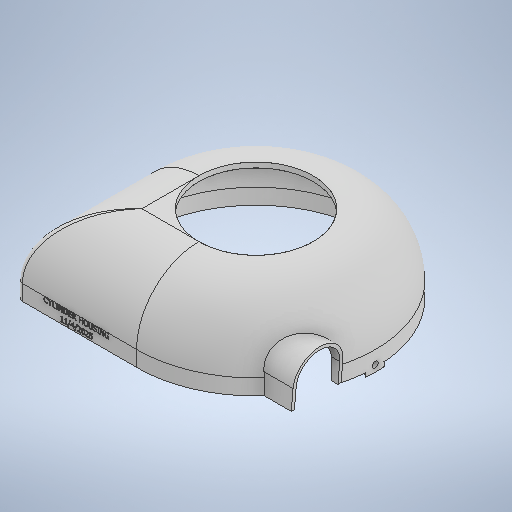
# Autodesk Inventor part: Cylinder Housing_cap_3
Saved by Autodesk Inventor 2025 (Build 290162000, 162)
## iProperties
Created: 2025-10-06
Part Number: Cylinder Housing_cap_3
Material: Generic
Document SubType Name: Modeling
Designer: mumin
Density: 1 g/cm^3
Appearance: Default
Author: mumin
Autodesk Inventor part; units mm, degrees
ref_plane "XZ Plane" through (0, 0, 0) normal (0, 1, 0) x (-1, 0, 0)
ref_plane "XY Plane" through (0, 0, 0) normal (0, 0, 1) x (1, 0, 0)
sketch "Sketch1" plane through (0, 0, 0) normal (0, 1, 0) x (-1, 0, 0)
  arc A0 (0, 115) -> (115, 0) centre (0, 0) ccw
  line L0 (115, 0) -> (115, 110)
  line L1 (110, 115) -> (0, 115)
  arc A1 (115, 110) -> (110, 115) centre (110, 110) ccw
  dimension "d0" = 230
  dimension "d1" = 5
  constraints: 4 end point, 4 point on circle, 2 centre point, 2 tangent, 1 coincident
  measures "d0" diameter of A0
  measures "d1" radius of A1
extrude "Base Shape & Wall" add sketch "Sketch1" along normal blind 75
fillet "Curved Edge" radius 60 4 edges at (81.3173, 75, -81.3173) (-115, 75, 55) (-113.5355, 75, 113.5355) (-55, 75, 115)
shell "Shell" thickness 4.9 removed faces 1 at (-52.6749, 0, -2.0856)
sketch "Sketch2" plane through (0, 75, 0) normal (0, 1, 0) x (1, 0, 0)
  point P0 (0, 0)
  point P1 (0, 0)
  constraints: 1 coincident
hole "Cylinder Hole" at (0, 75, 0) direction (0, -1, 0) diameter 109.9 end through all
sketch "Sketch3" plane through (0, 0, 0) normal (0, -1, 0) x (1, 0, 0)
  arc A0 (-115, 0) -> (0, 115) centre (0, 0) ccw projected
  line L0 (0, 55) -> (0, 110.1) projected
  line L1 (-110.1, 0) -> (-55, 0) projected
  arc A1 (-110.1, 0) -> (0, 110.1) centre (0, 0) ccw projected
  line L2 (114.6551, 8.9) -> (109.9418, 5.9)
  line L3 (109.9418, -5.9) -> (114.6551, -8.9)
  line L4 (-199.1076, 0) -> (222.9249, 0) projected
  arc A2 (-55, 0) -> (0, 55) centre (0, 0) ccw projected
  dimension "d13" = 5.9
  dimension "d14" = 8.9
  constraints: 4 end point, 4 point on circle, 2 symmetric about line
  measures "d13" distance from line of L4 L2.end
  measures "d14" distance from line of L4 L2.start
extrude "Front Tab" add sketch "Sketch3" along normal blind 4 contours L3 A1 L4 A0 | L4 A1 L2 A0 picked at (113.1479, -6.9122)
sketch "Sketch4" plane through (0, 0, 0) normal (1, 0, 0) x (0, 1, 0)
  line L0 (0, 0) -> (15, 0) projected
  circle A0 centre (2.5, 0) radius 2.75
  line L1 (-4, 8.9) -> (-4, -8.9) projected
  dimension "d17" = 5.5
  dimension "d18" = 6.5
  constraints: 1 centre point, 1 point on line
  measures "d17" diameter of A0
  measures "d18" distance from line of L1 A0.centre
extrude "Bolt Hole" cut sketch "Sketch4" along normal through all
sketch "Sketch5" plane through (0, 0, 0) normal (0, 0, 1) x (1, 0, 0)
  line L0 (-110.1, 0) -> (-108.0437, 0)
  line L1 (-110.1, 0) -> (-110.1, 15) projected
  line L2 (-110.1, 0) -> (-110.1, 10.1)
  line L3 (-110.1, 10.1) -> (-113.1, 10.1)
  line L4 (-113.1, 10.1) -> (-110.1, 0)
  line L5 (-109.0719, 10.1) -> (-109.0719, 0)
  line L6 (-110.1, 10.1) -> (-109.0719, 10.1)
  point P0 (0, 0)
  point P1 (0, 15)
  dimension "d43" = 10.1
  dimension "d44" = 3
  constraints: 12 end point, 2 horizontal, 1 midpoint, 1 perpendicular, 1 point on line
  measures "d43" distance of L0.start L2.end
  measures "d44" distance of L2.end L3.end
extrude "Hinge Tab Recess" cut sketch "Sketch5" along normal mid plane 15
sketch "Sketch6" plane through (0, 0, 0) normal (1, 0, 0) x (0, 1, 0)
  arc A0 (20, 32.226) -> (20, 74.226) centre (20, 53.226) ccw
  line L0 (0, 8.9) -> (0, 115) projected
  line L1 (20, 74.226) -> (0, 74.226)
  line L2 (0, 74.226) -> (0, 32.226)
  line L3 (0, 32.226) -> (20, 32.226)
  point P0 (0, 0)
  dimension "d25" = 42
  dimension "d26" = 53.226
  dimension "d27" = 20
  constraints: 6 end point, 2 point on circle, 1 centre point, 1 horizontal, 1 parallel, 1 perpendicular, 1 point on line
  measures "d25" diameter of A0
  measures "d26" vertical distance of point (0, 0) A0.centre
  measures "d27" distance from line of L0 A0.centre
extrude "LV Hole" cut sketch "Sketch6" along normal through all
ref_plane "Work Plane1" through (115, 0, 0) normal (1, 0, 0) x (0, 1, 0)
sketch "Sketch8" plane through (115, 0, 0) normal (1, 0, 0) x (0, 1, 0)
  spline S0 degree 5 poles (20, 74.226) (21.7452, 74.226) (23.5079, 74.045) (25.2552, 73.6747) (26.9529, 73.1202) (29.9438, 71.784) (31.2609, 71.0468) (32.4954, 70.2012) (33.6326, 69.2644) (35.8574, 67.094) (36.9093, 65.8358) (37.811, 64.5157) (38.5629, 63.1597) (39.9244, 60.1101) (40.4634, 58.4091) (40.8112, 56.7153) (40.9848, 55.0472) (41.0281, 50.1315) (40.4151, 46.9848) (39.2704, 44.0382) (37.5933, 41.2886) (34.2813, 37.7546) (33.1162, 36.7127) (31.8193, 35.7519) (30.3873, 34.8935) (28.01, 33.793) (27.1625, 33.4531) (26.2801, 33.1539) (25.3653, 32.9001) (23.9884, 32.6034) (23.5482, 32.5207) (23.1027, 32.4491) (22.6524, 32.3892) (21.7638, 32.2956) (21.3262, 32.261) (20.8833, 32.2376) (20.4431, 32.226) (20, 32.226) knots 0 0 0 0 0 0 0.115277 0.115277 0.115277 0.115277 0.213785 0.213785 0.213785 0.213785 0.327655 0.327655 0.327655 0.327655 0.466839 0.466839 0.466839 0.466839 0.745876 0.745876 0.745876 0.745876 0.873844 0.873844 0.873844 0.873844 0.940211 0.940211 0.940211 0.940211 0.970786 0.970786 0.970786 0.970786 1 1 1 1 1 1 projected
  line L0 (15, 74.226) -> (20, 74.226) projected
  line L1 (0, 74.226) -> (15, 74.226) projected
  line L2 (20, 32.226) -> (15, 32.226) projected
  line L3 (15, 32.226) -> (0, 32.226) projected
  line L4 (0, 29.226) -> (15, 29.226)
  line L5 (15, 29.226) -> (20, 29.226)
  line L6 (20, 77.226) -> (15, 77.226)
  line L7 (15, 77.226) -> (0, 77.226)
  line L8 (0, 77.226) -> (0, 74.226)
  line L9 (0, 0) -> (0, 110) projected
  line L10 (0, 32.226) -> (0, 29.226)
  spline S1 degree 5 poles (20, 29.226) (24.9777, 29.2263) (29.9563, 30.5154) (34.4863, 33.1008) (41.4168, 40.0057) (44.3283, 49.2848) (44.6352, 53.9403) (42.8551, 64.1602) (36.1874, 72.3028) (31.2207, 75.5896) (25.6093, 77.2254) (20, 77.226) knots 0 0 0 0 0 0 0.330105 0.330105 0.330105 0.628 0.628 0.628 1 1 1 1 1 1
  dimension "d38" = 3
  constraints: 12 end point, 2 collinear, 2 parallel, 2 vertical alignment, 4 other
extrude "LV Hood" add sketch "Sketch8" against normal up to surface contours L0 L1 L8 L7 L6 S1 L5 L4 L9 L3 L2 S0
sketch "Sketch9" plane through (115, 0, 77.226) normal (0, 0, 1) x (1, 0, 0)
  line L0 (-3.7757, 15) -> (-3.7757, 0) projected
  line L1 (0, 20) -> (-3.9915, 20) projected
  line L2 (0, 0) -> (0, 20) projected
  line L3 (0, 0) -> (-3.7757, 0) projected
  line L4 (0, 20) -> (0, 44) projected
  line L5 (-3.7757, 0) -> (0, 44)
  line L6 (0, 44) -> (0, 0)
  point P0 (-115, 0)
  constraints: 4 end point, 1 collinear, 1 other
extrude "Hood Slant Cut" cut sketch "Sketch9" against normal up to surface (48 mm away)
fillet "Fillet2" radius 0.2 1 edges at (-113.1, 10.1, 0)
sketch "Sketch10" plane through (-110, 0, 115) normal (0, 0, 1) x (1, 0, 0)
  line L0 (20.3517, 14.9708) -> (83.5486, 14.9708) construction
  line L1 (83.5486, 14.9708) -> (83.5486, 0.5472) construction
  line L2 (83.5486, 0.5472) -> (20.3517, 0.5472) construction
  line L3 (20.3517, 0.5472) -> (20.3517, 14.9708) construction
  spline S0 degree 2 poles (22.8112, 9.7763) (22.325, 9.7763) (21.5024, 10.1045) (21.2026, 10.4327) knots 0 0 0 1 2 2 2
  spline S1 degree 2 poles (21.2026, 10.4327) (20.9028, 10.7569) (20.5746, 11.7293) (20.5746, 12.3614) knots 0 0 0 1 2 2 2
  spline S2 degree 2 poles (20.5746, 12.3614) (20.5746, 12.9895) (20.8947, 13.9214) (21.1985, 14.2658) knots 0 0 0 1 2 2 2
  spline S3 degree 2 poles (21.1985, 14.2658) (21.4984, 14.6021) (22.3169, 14.9546) (22.8233, 14.9546) knots 0 0 0 1 2 2 2
  spline S4 degree 2 poles (22.8233, 14.9546) (23.0746, 14.9546) (23.5162, 14.8817) (23.7026, 14.825) knots 0 0 0 1 2 2 2
  spline S5 degree 2 poles (23.7026, 14.825) (23.8647, 14.7723) (24.201, 14.6224) (24.3671, 14.5332) knots 0 0 0 1 2 2 2
  line L4 (24.3671, 14.5332) -> (24.3671, 13.7309)
  line L5 (24.3671, 13.7309) -> (24.3144, 13.7309)
  spline S6 degree 2 poles (24.3144, 13.7309) (24.2253, 13.812) (23.9498, 14.0389) (23.7512, 14.1483) knots 0 0 0 1 2 2 2
  spline S7 degree 2 poles (23.7512, 14.1483) (23.5608, 14.2536) (23.111, 14.3873) (22.8193, 14.3873) knots 0 0 0 1 2 2 2
  spline S8 degree 2 poles (22.8193, 14.3873) (22.4992, 14.3873) (21.9279, 14.124) (21.7131, 13.8728) knots 0 0 0 1 2 2 2
  spline S9 degree 2 poles (21.7131, 13.8728) (21.5024, 13.6175) (21.2674, 12.8436) (21.2674, 12.3614) knots 0 0 0 1 2 2 2
  spline S10 degree 2 poles (21.2674, 12.3614) (21.2674, 11.8468) (21.5146, 11.1053) (21.7293, 10.8501) knots 0 0 0 1 2 2 2
  spline S11 degree 2 poles (21.7293, 10.8501) (21.94, 10.6029) (22.5032, 10.3517) (22.8193, 10.3517) knots 0 0 0 1 2 2 2
  spline S12 degree 2 poles (22.8193, 10.3517) (23.107, 10.3517) (23.5972, 10.4935) (23.7877, 10.5989) knots 0 0 0 1 2 2 2
  spline S13 degree 2 poles (23.7877, 10.5989) (23.97, 10.7042) (24.2415, 10.923) (24.3185, 11) knots 0 0 0 1 2 2 2
  line L6 (24.3185, 11) -> (24.3671, 11)
  line L7 (24.3671, 11) -> (24.3671, 10.2058)
  spline S14 degree 2 poles (24.3671, 10.2058) (24.201, 10.1288) (23.9092, 9.987) (23.7026, 9.9222) knots 0 0 0 1 2 2 2
  spline S15 degree 2 poles (23.7026, 9.9222) (23.4838, 9.8493) (23.111, 9.7763) (22.8112, 9.7763) knots 0 0 0 1 2 2 2
  line L8 (28.4878, 14.8655) -> (26.7982, 12.0778)
  line L9 (26.7982, 12.0778) -> (26.7982, 9.8655)
  line L10 (26.7982, 9.8655) -> (26.1337, 9.8655)
  line L11 (26.1337, 9.8655) -> (26.1337, 12.0089)
  line L12 (26.1337, 12.0089) -> (24.4441, 14.8655)
  line L13 (24.4441, 14.8655) -> (25.1815, 14.8655)
  line L14 (25.1815, 14.8655) -> (26.4741, 12.6653)
  line L15 (26.4741, 12.6653) -> (27.7828, 14.8655)
  line L16 (27.7828, 14.8655) -> (28.4878, 14.8655)
  line L17 (31.8468, 9.8655) -> (28.9498, 9.8655)
  line L18 (28.9498, 9.8655) -> (28.9498, 14.8655)
  line L19 (28.9498, 14.8655) -> (29.6143, 14.8655)
  line L20 (29.6143, 14.8655) -> (29.6143, 10.457)
  line L21 (29.6143, 10.457) -> (31.8468, 10.457)
  line L22 (31.8468, 10.457) -> (31.8468, 9.8655)
  line L23 (34.1118, 9.8655) -> (32.175, 9.8655)
  line L24 (32.175, 9.8655) -> (32.175, 10.376)
  line L25 (32.175, 10.376) -> (32.8112, 10.376)
  line L26 (32.8112, 10.376) -> (32.8112, 14.3549)
  line L27 (32.8112, 14.3549) -> (32.175, 14.3549)
  line L28 (32.175, 14.3549) -> (32.175, 14.8655)
  line L29 (32.175, 14.8655) -> (34.1118, 14.8655)
  line L30 (34.1118, 14.8655) -> (34.1118, 14.3549)
  line L31 (34.1118, 14.3549) -> (33.4757, 14.3549)
  line L32 (33.4757, 14.3549) -> (33.4757, 10.376)
  line L33 (33.4757, 10.376) -> (34.1118, 10.376)
  line L34 (34.1118, 10.376) -> (34.1118, 9.8655)
  line L35 (38.5122, 9.8655) -> (37.7666, 9.8655)
  line L36 (37.7666, 9.8655) -> (35.5543, 14.1767)
  line L37 (35.5543, 14.1767) -> (35.5543, 9.8655)
  line L38 (35.5543, 9.8655) -> (34.9344, 9.8655)
  line L39 (34.9344, 9.8655) -> (34.9344, 14.8655)
  line L40 (34.9344, 14.8655) -> (35.8784, 14.8655)
  line L41 (35.8784, 14.8655) -> (37.8922, 10.9068)
  line L42 (37.8922, 10.9068) -> (37.8922, 14.8655)
  line L43 (37.8922, 14.8655) -> (38.5122, 14.8655)
  line L44 (38.5122, 14.8655) -> (38.5122, 9.8655)
  spline S16 degree 2 poles (43.4676, 12.3614) (43.4676, 11.6767) (42.9125, 10.5745) (42.4465, 10.2666) knots 0 0 0 1 2 2 2
  spline S17 degree 2 poles (42.4465, 10.2666) (42.0656, 10.0275) (41.2836, 9.8655) (40.6759, 9.8655) knots 0 0 0 1 2 2 2
  line L45 (40.6759, 9.8655) -> (39.5251, 9.8655)
  line L46 (39.5251, 9.8655) -> (39.5251, 14.8655)
  line L47 (39.5251, 14.8655) -> (40.6637, 14.8655)
  spline S18 degree 2 poles (40.6637, 14.8655) (41.3687, 14.8655) (42.171, 14.6548) (42.4546, 14.4684) knots 0 0 0 1 2 2 2
  spline S19 degree 2 poles (42.4546, 14.4684) (42.9368, 14.1483) (43.4676, 13.0908) (43.4676, 12.3614) knots 0 0 0 1 2 2 2
  spline S20 degree 2 poles (42.7747, 12.3695) (42.7747, 12.9449) (42.3938, 13.7593) (42.017, 13.9903) knots 0 0 0 1 2 2 2
  spline S21 degree 2 poles (42.017, 13.9903) (41.7496, 14.1483) (41.1459, 14.2901) (40.6961, 14.2901) knots 0 0 0 1 2 2 2
  line L48 (40.6961, 14.2901) -> (40.1896, 14.2901)
  line L49 (40.1896, 14.2901) -> (40.1896, 10.4408)
  line L50 (40.1896, 10.4408) -> (40.6961, 10.4408)
  spline S22 degree 2 poles (40.6961, 10.4408) (41.1378, 10.4408) (41.8063, 10.5826) (42.0778, 10.7731) knots 0 0 0 1 2 2 2
  spline S23 degree 2 poles (42.0778, 10.7731) (42.4263, 11.0081) (42.7747, 11.7861) (42.7747, 12.3695) knots 0 0 0 1 2 2 2
  line L51 (44.1888, 9.8655) -> (44.1888, 14.8655)
  line L52 (44.1888, 14.8655) -> (47.3169, 14.8655)
  line L53 (47.3169, 14.8655) -> (47.3169, 14.2739)
  line L54 (47.3169, 14.2739) -> (44.8533, 14.2739)
  line L55 (44.8533, 14.2739) -> (44.8533, 12.9044)
  line L56 (44.8533, 12.9044) -> (47.1507, 12.9044)
  line L57 (47.1507, 12.9044) -> (47.1507, 12.3128)
  line L58 (47.1507, 12.3128) -> (44.8533, 12.3128)
  line L59 (44.8533, 12.3128) -> (44.8533, 10.457)
  line L60 (44.8533, 10.457) -> (47.3169, 10.457)
  line L61 (47.3169, 10.457) -> (47.3169, 9.8655)
  line L62 (47.3169, 9.8655) -> (44.1888, 9.8655)
  line L63 (51.9157, 9.8655) -> (51.0527, 9.8655)
  line L64 (51.0527, 9.8655) -> (49.4725, 11.8549)
  line L65 (49.4725, 11.8549) -> (48.7107, 11.8549)
  line L66 (48.7107, 11.8549) -> (48.7107, 9.8655)
  line L67 (48.7107, 9.8655) -> (48.0462, 9.8655)
  line L68 (48.0462, 9.8655) -> (48.0462, 14.8655)
  line L69 (48.0462, 14.8655) -> (49.3347, 14.8655)
  spline S24 degree 2 poles (49.3347, 14.8655) (49.7642, 14.8655) (50.3436, 14.7723) (50.607, 14.6021) knots 0 0 0 1 2 2 2
  spline S25 degree 2 poles (50.607, 14.6021) (50.8703, 14.4319) (51.1742, 13.9011) (51.1742, 13.5081) knots 0 0 0 1 2 2 2
  spline S26 degree 2 poles (51.1742, 13.5081) (51.1742, 12.9611) (50.6151, 12.2196) (50.137, 12.0413) knots 0 0 0 1 2 2 2
  line L70 (50.137, 12.0413) -> (51.9157, 9.8655)
  spline S27 degree 2 poles (50.4814, 13.4554) (50.4814, 13.6742) (50.3274, 14.0105) (50.1653, 14.1199) knots 0 0 0 1 2 2 2
  spline S28 degree 2 poles (50.1653, 14.1199) (50.0235, 14.2131) (49.6467, 14.2901) (49.3712, 14.2901) knots 0 0 0 1 2 2 2
  line L71 (49.3712, 14.2901) -> (48.7107, 14.2901)
  line L72 (48.7107, 14.2901) -> (48.7107, 12.41)
  line L73 (48.7107, 12.41) -> (49.2942, 12.41)
  spline S29 degree 2 poles (49.2942, 12.41) (49.5819, 12.41) (50.0397, 12.5113) (50.1977, 12.6694) knots 0 0 0 1 2 2 2
  spline S30 degree 2 poles (50.1977, 12.6694) (50.3436, 12.8071) (50.4814, 13.1961) (50.4814, 13.4554) knots 0 0 0 1 2 2 2
  line L74 (58.0908, 9.8655) -> (57.4263, 9.8655)
  line L75 (57.4263, 9.8655) -> (57.4263, 12.3128)
  line L76 (57.4263, 12.3128) -> (55.1248, 12.3128)
  line L77 (55.1248, 12.3128) -> (55.1248, 9.8655)
  line L78 (55.1248, 9.8655) -> (54.4603, 9.8655)
  line L79 (54.4603, 9.8655) -> (54.4603, 14.8655)
  line L80 (54.4603, 14.8655) -> (55.1248, 14.8655)
  line L81 (55.1248, 14.8655) -> (55.1248, 12.9044)
  line L82 (55.1248, 12.9044) -> (57.4263, 12.9044)
  line L83 (57.4263, 12.9044) -> (57.4263, 14.8655)
  line L84 (57.4263, 14.8655) -> (58.0908, 14.8655)
  line L85 (58.0908, 14.8655) -> (58.0908, 9.8655)
  spline S31 degree 2 poles (62.641, 14.2942) (62.9246, 13.9619) (63.2407, 12.9895) (63.2407, 12.3655) knots 0 0 0 1 2 2 2
  spline S32 degree 2 poles (63.2407, 12.3655) (63.2407, 11.7577) (62.9327, 10.7731) (62.641, 10.4408) knots 0 0 0 1 2 2 2
  spline S33 degree 2 poles (62.641, 10.4408) (62.3331, 10.0924) (61.5186, 9.7601) (61.0284, 9.7601) knots 0 0 0 1 2 2 2
  spline S34 degree 2 poles (61.0284, 9.7601) (60.5219, 9.7601) (59.7115, 10.1045) (59.4157, 10.4408) knots 0 0 0 1 2 2 2
  spline S35 degree 2 poles (59.4157, 10.4408) (59.128, 10.7731) (58.8201, 11.7496) (58.8201, 12.3655) knots 0 0 0 1 2 2 2
  spline S36 degree 2 poles (58.8201, 12.3655) (58.8201, 12.9935) (59.1321, 13.9497) (59.4198, 14.2942) knots 0 0 0 1 2 2 2
  spline S37 degree 2 poles (59.4198, 14.2942) (59.7115, 14.6264) (60.5259, 14.9708) (61.0284, 14.9708) knots 0 0 0 1 2 2 2
  spline S38 degree 2 poles (61.0284, 14.9708) (61.5389, 14.9708) (62.3574, 14.6143) (62.641, 14.2942) knots 0 0 0 1 2 2 2
  spline S39 degree 2 poles (62.5478, 12.3655) (62.5478, 12.8598) (62.3331, 13.6256) (62.1386, 13.8768) knots 0 0 0 1 2 2 2
  spline S40 degree 2 poles (62.1386, 13.8768) (61.94, 14.1361) (61.3809, 14.3955) (61.0324, 14.3955) knots 0 0 0 1 2 2 2
  spline S41 degree 2 poles (61.0324, 14.3955) (60.6718, 14.3955) (60.1289, 14.1442) (59.9222, 13.8768) knots 0 0 0 1 2 2 2
  spline S42 degree 2 poles (59.9222, 13.8768) (59.7237, 13.6215) (59.513, 12.8517) (59.513, 12.3655) knots 0 0 0 1 2 2 2
  spline S43 degree 2 poles (59.513, 12.3655) (59.513, 11.3809) (60.3395, 10.3355) (61.0324, 10.3355) knots 0 0 0 1 2 2 2
  spline S44 degree 2 poles (61.0324, 10.3355) (61.7253, 10.3355) (62.5478, 11.3809) (62.5478, 12.3655) knots 0 0 0 1 2 2 2
  spline S45 degree 2 poles (65.7164, 9.7601) (65.2747, 9.7601) (64.6183, 9.9911) (64.3874, 10.222) knots 0 0 0 1 2 2 2
  spline S46 degree 2 poles (64.3874, 10.222) (64.124, 10.4814) (63.9092, 11.2107) (63.9092, 11.7455) knots 0 0 0 1 2 2 2
  line L86 (63.9092, 11.7455) -> (63.9092, 14.8655)
  line L87 (63.9092, 14.8655) -> (64.5737, 14.8655)
  line L88 (64.5737, 14.8655) -> (64.5737, 11.7455)
  spline S47 degree 2 poles (64.5737, 11.7455) (64.5737, 11.3971) (64.6629, 10.9271) (64.7885, 10.7366) knots 0 0 0 1 2 2 2
  spline S48 degree 2 poles (64.7885, 10.7366) (64.9222, 10.534) (65.3841, 10.3274) (65.7164, 10.3274) knots 0 0 0 1 2 2 2
  spline S49 degree 2 poles (65.7164, 10.3274) (66.0284, 10.3274) (66.5146, 10.534) (66.6483, 10.7366) knots 0 0 0 1 2 2 2
  spline S50 degree 2 poles (66.6483, 10.7366) (66.7739, 10.9271) (66.8631, 11.393) (66.8631, 11.7293) knots 0 0 0 1 2 2 2
  line L89 (66.8631, 11.7293) -> (66.8631, 14.8655)
  line L90 (66.8631, 14.8655) -> (67.5276, 14.8655)
  line L91 (67.5276, 14.8655) -> (67.5276, 11.7455)
  spline S51 degree 2 poles (67.5276, 11.7455) (67.5276, 11.2228) (67.3169, 10.4773) (67.0494, 10.222) knots 0 0 0 1 2 2 2
  spline S52 degree 2 poles (67.0494, 10.222) (66.8104, 9.987) (66.1783, 9.7601) (65.7164, 9.7601) knots 0 0 0 1 2 2 2
  spline S53 degree 2 poles (69.8736, 9.7763) (69.3306, 9.7763) (68.5689, 10.0032) (68.2326, 10.1653) knots 0 0 0 1 2 2 2
  line L92 (68.2326, 10.1653) -> (68.2326, 11)
  line L93 (68.2326, 11) -> (68.2812, 11)
  spline S54 degree 2 poles (68.2812, 11) (68.6094, 10.6921) (69.44, 10.3517) (69.825, 10.3517) knots 0 0 0 1 2 2 2
  spline S55 degree 2 poles (69.825, 10.3517) (70.376, 10.3517) (70.9392, 10.8096) (70.9392, 11.1864) knots 0 0 0 1 2 2 2
  spline S56 degree 2 poles (70.9392, 11.1864) (70.9392, 11.4862) (70.6434, 11.859) (70.3233, 11.9522) knots 0 0 0 1 2 2 2
  spline S57 degree 2 poles (70.3233, 11.9522) (70.0924, 12.017) (69.7075, 12.1062) (69.4198, 12.1791) knots 0 0 0 1 2 2 2
  spline S58 degree 2 poles (69.4198, 12.1791) (69.1605, 12.248) (68.7512, 12.4546) (68.5932, 12.6207) knots 0 0 0 1 2 2 2
  spline S59 degree 2 poles (68.5932, 12.6207) (68.4392, 12.7869) (68.269, 13.2326) (68.269, 13.5243) knots 0 0 0 1 2 2 2
  spline S60 degree 2 poles (68.269, 13.5243) (68.269, 14.1321) (69.2172, 14.9546) (69.9506, 14.9546) knots 0 0 0 1 2 2 2
  spline S61 degree 2 poles (69.9506, 14.9546) (70.372, 14.9546) (71.1175, 14.7885) (71.4376, 14.6305) knots 0 0 0 1 2 2 2
  line L94 (71.4376, 14.6305) -> (71.4376, 13.8363)
  line L95 (71.4376, 13.8363) -> (71.389, 13.8363)
  spline S62 degree 2 poles (71.389, 13.8363) (71.1499, 14.0551) (70.4044, 14.3792) (69.9951, 14.3792) knots 0 0 0 1 2 2 2
  spline S63 degree 2 poles (69.9951, 14.3792) (69.5332, 14.3792) (68.9619, 13.9457) (68.9619, 13.5932) knots 0 0 0 1 2 2 2
  spline S64 degree 2 poles (68.9619, 13.5932) (68.9619, 13.2771) (69.2982, 12.9003) (69.6143, 12.8152) knots 0 0 0 1 2 2 2
  spline S65 degree 2 poles (69.6143, 12.8152) (69.825, 12.7585) (70.4368, 12.6126) (70.6394, 12.5519) knots 0 0 0 1 2 2 2
  spline S66 degree 2 poles (70.6394, 12.5519) (71.154, 12.3938) (71.6321, 11.7577) (71.6321, 11.2917) knots 0 0 0 1 2 2 2
  spline S67 degree 2 poles (71.6321, 11.2917) (71.6321, 10.9959) (71.393, 10.4287) (71.1783, 10.2301) knots 0 0 0 1 2 2 2
  spline S68 degree 2 poles (71.1783, 10.2301) (70.9392, 10.0113) (70.3314, 9.7763) (69.8736, 9.7763) knots 0 0 0 1 2 2 2
  line L96 (74.0511, 9.8655) -> (72.1143, 9.8655)
  line L97 (72.1143, 9.8655) -> (72.1143, 10.376)
  line L98 (72.1143, 10.376) -> (72.7504, 10.376)
  line L99 (72.7504, 10.376) -> (72.7504, 14.3549)
  line L100 (72.7504, 14.3549) -> (72.1143, 14.3549)
  line L101 (72.1143, 14.3549) -> (72.1143, 14.8655)
  line L102 (72.1143, 14.8655) -> (74.0511, 14.8655)
  line L103 (74.0511, 14.8655) -> (74.0511, 14.3549)
  line L104 (74.0511, 14.3549) -> (73.4149, 14.3549)
  line L105 (73.4149, 14.3549) -> (73.4149, 10.376)
  line L106 (73.4149, 10.376) -> (74.0511, 10.376)
  line L107 (74.0511, 10.376) -> (74.0511, 9.8655)
  line L108 (78.4514, 9.8655) -> (77.7058, 9.8655)
  line L109 (77.7058, 9.8655) -> (75.4935, 14.1767)
  line L110 (75.4935, 14.1767) -> (75.4935, 9.8655)
  line L111 (75.4935, 9.8655) -> (74.8736, 9.8655)
  line L112 (74.8736, 9.8655) -> (74.8736, 14.8655)
  line L113 (74.8736, 14.8655) -> (75.8177, 14.8655)
  line L114 (75.8177, 14.8655) -> (77.8314, 10.9068)
  line L115 (77.8314, 10.9068) -> (77.8314, 14.8655)
  line L116 (77.8314, 14.8655) -> (78.4514, 14.8655)
  line L117 (78.4514, 14.8655) -> (78.4514, 9.8655)
  spline S69 degree 2 poles (81.5592, 9.7682) (81.0284, 9.7682) (80.1491, 10.0924) (79.8331, 10.4206) knots 0 0 0 1 2 2 2
  spline S70 degree 2 poles (79.8331, 10.4206) (79.517, 10.7528) (79.1807, 11.7334) (79.1807, 12.3695) knots 0 0 0 1 2 2 2
  spline S71 degree 2 poles (79.1807, 12.3695) (79.1807, 12.9732) (79.5211, 13.9295) (79.8371, 14.2698) knots 0 0 0 1 2 2 2
  spline S72 degree 2 poles (79.8371, 14.2698) (80.141, 14.598) (81.0324, 14.9546) (81.5632, 14.9546) knots 0 0 0 1 2 2 2
  spline S73 degree 2 poles (81.5632, 14.9546) (81.8185, 14.9546) (82.2804, 14.8817) (82.4911, 14.8168) knots 0 0 0 1 2 2 2
  spline S74 degree 2 poles (82.4911, 14.8168) (82.6613, 14.7682) (83.0746, 14.5899) (83.2002, 14.5251) knots 0 0 0 1 2 2 2
  line L118 (83.2002, 14.5251) -> (83.2002, 13.7228)
  line L119 (83.2002, 13.7228) -> (83.1434, 13.7228)
  spline S75 degree 2 poles (83.1434, 13.7228) (83.0178, 13.8322) (82.7545, 14.0308) (82.5113, 14.1442) knots 0 0 0 1 2 2 2
  spline S76 degree 2 poles (82.5113, 14.1442) (82.3088, 14.2455) (81.7861, 14.3792) (81.4862, 14.3792) knots 0 0 0 1 2 2 2
  spline S77 degree 2 poles (81.4862, 14.3792) (80.765, 14.3792) (79.8736, 13.2933) (79.8736, 12.3898) knots 0 0 0 1 2 2 2
  spline S78 degree 2 poles (79.8736, 12.3898) (79.8736, 11.8873) (80.1086, 11.1337) (80.3314, 10.8744) knots 0 0 0 1 2 2 2
  spline S79 degree 2 poles (80.3314, 10.8744) (80.5462, 10.6151) (81.154, 10.3436) (81.5348, 10.3436) knots 0 0 0 1 2 2 2
  spline S80 degree 2 poles (81.5348, 10.3436) (81.8144, 10.3436) (82.3736, 10.4246) (82.564, 10.5057) knots 0 0 0 1 2 2 2
  line L120 (82.564, 10.5057) -> (82.564, 11.7982)
  line L121 (82.564, 11.7982) -> (81.4052, 11.7982)
  line L122 (81.4052, 11.7982) -> (81.4052, 12.3817)
  line L123 (81.4052, 12.3817) -> (83.2204, 12.3817)
  line L124 (83.2204, 12.3817) -> (83.2204, 10.1977)
  spline S81 degree 2 poles (83.2204, 10.1977) (83.0948, 10.141) (82.6653, 9.9668) (82.483, 9.9141) knots 0 0 0 1 2 2 2
  spline S82 degree 2 poles (82.483, 9.9141) (82.2358, 9.8412) (81.8387, 9.7682) (81.5592, 9.7682) knots 0 0 0 1 2 2 2
  line L125 (39.3853, 1.6331) -> (36.9461, 1.6331)
  line L126 (36.9461, 1.6331) -> (36.9461, 2.1436)
  line L127 (36.9461, 2.1436) -> (37.8537, 2.1436)
  line L128 (37.8537, 2.1436) -> (37.8537, 5.4945)
  line L129 (37.8537, 5.4945) -> (36.9461, 5.4945)
  line L130 (36.9461, 5.4945) -> (36.9461, 5.9524)
  spline S83 degree 2 poles (36.9461, 5.9524) (37.4607, 5.9524) (37.9469, 6.2441) (37.9793, 6.6493) knots 0 0 0 1 2 2 2
  line L131 (37.9793, 6.6493) -> (38.498, 6.6493)
  line L132 (38.498, 6.6493) -> (38.498, 2.1436)
  line L133 (38.498, 2.1436) -> (39.3853, 2.1436)
  line L134 (39.3853, 2.1436) -> (39.3853, 1.6331)
  line L135 (43.1374, 1.6331) -> (40.6981, 1.6331)
  line L136 (40.6981, 1.6331) -> (40.6981, 2.1436)
  line L137 (40.6981, 2.1436) -> (41.6058, 2.1436)
  line L138 (41.6058, 2.1436) -> (41.6058, 5.4945)
  line L139 (41.6058, 5.4945) -> (40.6981, 5.4945)
  line L140 (40.6981, 5.4945) -> (40.6981, 5.9524)
  spline S84 degree 2 poles (40.6981, 5.9524) (41.2127, 5.9524) (41.699, 6.2441) (41.7314, 6.6493) knots 0 0 0 1 2 2 2
  line L141 (41.7314, 6.6493) -> (42.25, 6.6493)
  line L142 (42.25, 6.6493) -> (42.25, 2.1436)
  line L143 (42.25, 2.1436) -> (43.1374, 2.1436)
  line L144 (43.1374, 2.1436) -> (43.1374, 1.6331)
  line L145 (46.1357, 6.856) -> (44.1787, 0.5472)
  line L146 (44.1787, 0.5472) -> (43.6114, 0.5472)
  line L147 (43.6114, 0.5472) -> (45.5604, 6.856)
  line L148 (45.5604, 6.856) -> (46.1357, 6.856)
  line L149 (49.904, 3.3511) -> (49.3084, 3.3511)
  line L150 (49.3084, 3.3511) -> (49.3084, 1.6331)
  line L151 (49.3084, 1.6331) -> (48.6641, 1.6331)
  line L152 (48.6641, 1.6331) -> (48.6641, 3.3511)
  line L153 (48.6641, 3.3511) -> (46.4558, 3.3511)
  line L154 (46.4558, 3.3511) -> (46.4558, 4.0561)
  line L155 (46.4558, 4.0561) -> (48.6925, 6.6331)
  line L156 (48.6925, 6.6331) -> (49.3084, 6.6331)
  line L157 (49.3084, 6.6331) -> (49.3084, 3.89)
  line L158 (49.3084, 3.89) -> (49.904, 3.89)
  line L159 (49.904, 3.89) -> (49.904, 3.3511)
  line L160 (48.6641, 3.89) -> (48.6641, 5.843)
  line L161 (48.6641, 5.843) -> (46.9826, 3.89)
  line L162 (46.9826, 3.89) -> (48.6641, 3.89)
  line L163 (52.5174, 6.856) -> (50.5604, 0.5472)
  line L164 (50.5604, 0.5472) -> (49.9931, 0.5472)
  line L165 (49.9931, 0.5472) -> (51.9421, 6.856)
  line L166 (51.9421, 6.856) -> (52.5174, 6.856)
  line L167 (56.1519, 1.6331) -> (53.0685, 1.6331)
  line L168 (53.0685, 1.6331) -> (53.0685, 2.3422)
  spline S85 degree 2 poles (53.0685, 2.3422) (53.4007, 2.6542) (53.9923, 3.2336) (54.2759, 3.5456) knots 0 0 0 1 2 2 2
  spline S86 degree 2 poles (54.2759, 3.5456) (54.8472, 4.1736) (55.2646, 4.9273) (55.2646, 5.3284) knots 0 0 0 1 2 2 2
  spline S87 degree 2 poles (55.2646, 5.3284) (55.2646, 5.5391) (55.1349, 5.8551) (55.0174, 5.9564) knots 0 0 0 1 2 2 2
  spline S88 degree 2 poles (55.0174, 5.9564) (54.8999, 6.0577) (54.592, 6.159) (54.4056, 6.159) knots 0 0 0 1 2 2 2
  spline S89 degree 2 poles (54.4056, 6.159) (54.2273, 6.159) (53.8626, 6.0699) (53.6965, 6.001) knots 0 0 0 1 2 2 2
  spline S90 degree 2 poles (53.6965, 6.001) (53.5547, 5.9443) (53.2913, 5.7822) (53.2103, 5.7255) knots 0 0 0 1 2 2 2
  line L169 (53.2103, 5.7255) -> (53.1738, 5.7255)
  line L170 (53.1738, 5.7255) -> (53.1738, 6.4386)
  spline S91 degree 2 poles (53.1738, 6.4386) (53.3805, 6.5399) (54.122, 6.7385) (54.4542, 6.7385) knots 0 0 0 1 2 2 2
  spline S92 degree 2 poles (54.4542, 6.7385) (55.1552, 6.7385) (55.9453, 5.997) (55.9453, 5.3649) knots 0 0 0 1 2 2 2
  spline S93 degree 2 poles (55.9453, 5.3649) (55.9453, 5.0691) (55.8075, 4.5748) (55.686, 4.3641) knots 0 0 0 1 2 2 2
  spline S94 degree 2 poles (55.686, 4.3641) (55.5644, 4.1453) (55.2119, 3.7158) (55.0174, 3.5091) knots 0 0 0 1 2 2 2
  spline S95 degree 2 poles (55.0174, 3.5091) (54.7014, 3.1647) (53.9275, 2.4273) (53.6965, 2.2125) knots 0 0 0 1 2 2 2
  line L171 (53.6965, 2.2125) -> (56.1519, 2.2125)
  line L172 (56.1519, 2.2125) -> (56.1519, 1.6331)
  spline S96 degree 2 poles (59.9323, 4.1331) (59.9323, 2.7879) (59.1503, 1.5278) (58.3359, 1.5278) knots 0 0 0 1 2 2 2
  spline S97 degree 2 poles (58.3359, 1.5278) (57.5093, 1.5278) (56.7354, 2.8122) (56.7354, 4.129) knots 0 0 0 1 2 2 2
  spline S98 degree 2 poles (56.7354, 4.129) (56.7354, 5.4824) (57.5174, 6.7344) (58.3359, 6.7344) knots 0 0 0 1 2 2 2
  spline S99 degree 2 poles (58.3359, 6.7344) (59.1584, 6.7344) (59.9323, 5.4378) (59.9323, 4.1331) knots 0 0 0 1 2 2 2
  spline S100 degree 2 poles (59.0733, 2.6096) (59.1706, 2.8568) (59.2516, 3.6185) (59.2516, 4.1331) knots 0 0 0 1 2 2 2
  spline S101 degree 2 poles (59.2516, 4.1331) (59.2516, 4.6477) (59.1706, 5.4054) (59.0693, 5.6607) knots 0 0 0 1 2 2 2
  spline S102 degree 2 poles (59.0693, 5.6607) (58.968, 5.9159) (58.6155, 6.1793) (58.3359, 6.1793) knots 0 0 0 1 2 2 2
  spline S103 degree 2 poles (58.3359, 6.1793) (58.0563, 6.1793) (57.6957, 5.9159) (57.5904, 5.6526) knots 0 0 0 1 2 2 2
  spline S104 degree 2 poles (57.5904, 5.6526) (57.4891, 5.3973) (57.4161, 4.6193) (57.4161, 4.129) knots 0 0 0 1 2 2 2
  spline S105 degree 2 poles (57.4161, 4.129) (57.4161, 3.6023) (57.481, 2.8973) (57.5863, 2.6218) knots 0 0 0 1 2 2 2
  spline S106 degree 2 poles (57.5863, 2.6218) (57.6836, 2.3624) (58.0442, 2.0829) (58.3359, 2.0829) knots 0 0 0 1 2 2 2
  spline S107 degree 2 poles (58.3359, 2.0829) (58.6114, 2.0829) (58.972, 2.3462) (59.0733, 2.6096) knots 0 0 0 1 2 2 2
  line L173 (63.656, 1.6331) -> (60.5725, 1.6331)
  line L174 (60.5725, 1.6331) -> (60.5725, 2.3422)
  spline S108 degree 2 poles (60.5725, 2.3422) (60.9048, 2.6542) (61.4964, 3.2336) (61.78, 3.5456) knots 0 0 0 1 2 2 2
  spline S109 degree 2 poles (61.78, 3.5456) (62.3513, 4.1736) (62.7686, 4.9273) (62.7686, 5.3284) knots 0 0 0 1 2 2 2
  spline S110 degree 2 poles (62.7686, 5.3284) (62.7686, 5.5391) (62.639, 5.8551) (62.5215, 5.9564) knots 0 0 0 1 2 2 2
  spline S111 degree 2 poles (62.5215, 5.9564) (62.404, 6.0577) (62.096, 6.159) (61.9096, 6.159) knots 0 0 0 1 2 2 2
  spline S112 degree 2 poles (61.9096, 6.159) (61.7314, 6.159) (61.3667, 6.0699) (61.2006, 6.001) knots 0 0 0 1 2 2 2
  spline S113 degree 2 poles (61.2006, 6.001) (61.0588, 5.9443) (60.7954, 5.7822) (60.7143, 5.7255) knots 0 0 0 1 2 2 2
  line L175 (60.7143, 5.7255) -> (60.6779, 5.7255)
  line L176 (60.6779, 5.7255) -> (60.6779, 6.4386)
  spline S114 degree 2 poles (60.6779, 6.4386) (60.8845, 6.5399) (61.626, 6.7385) (61.9583, 6.7385) knots 0 0 0 1 2 2 2
  spline S115 degree 2 poles (61.9583, 6.7385) (62.6592, 6.7385) (63.4494, 5.997) (63.4494, 5.3649) knots 0 0 0 1 2 2 2
  spline S116 degree 2 poles (63.4494, 5.3649) (63.4494, 5.0691) (63.3116, 4.5748) (63.19, 4.3641) knots 0 0 0 1 2 2 2
  spline S117 degree 2 poles (63.19, 4.3641) (63.0685, 4.1453) (62.716, 3.7158) (62.5215, 3.5091) knots 0 0 0 1 2 2 2
  spline S118 degree 2 poles (62.5215, 3.5091) (62.2054, 3.1647) (61.4315, 2.4273) (61.2006, 2.2125) knots 0 0 0 1 2 2 2
  line L177 (61.2006, 2.2125) -> (63.656, 2.2125)
  line L178 (63.656, 2.2125) -> (63.656, 1.6331)
  spline S119 degree 2 poles (67.3554, 3.2214) (67.3554, 2.8608) (67.1244, 2.2449) (66.9137, 2.018) knots 0 0 0 1 2 2 2
  spline S120 degree 2 poles (66.9137, 2.018) (66.703, 1.7911) (66.075, 1.5278) (65.686, 1.5278) knots 0 0 0 1 2 2 2
  spline S121 degree 2 poles (65.686, 1.5278) (65.3294, 1.5278) (64.6325, 1.6858) (64.3772, 1.8114) knots 0 0 0 1 2 2 2
  line L179 (64.3772, 1.8114) -> (64.3772, 2.5205)
  line L180 (64.3772, 2.5205) -> (64.4259, 2.5205)
  spline S122 degree 2 poles (64.4259, 2.5205) (64.5028, 2.4637) (64.7905, 2.3179) (64.9648, 2.253) knots 0 0 0 1 2 2 2
  spline S123 degree 2 poles (64.9648, 2.253) (65.1633, 2.1842) (65.4915, 2.1072) (65.6981, 2.1072) knots 0 0 0 1 2 2 2
  spline S124 degree 2 poles (65.6981, 2.1072) (65.9007, 2.1072) (66.2816, 2.253) (66.4194, 2.4111) knots 0 0 0 1 2 2 2
  spline S125 degree 2 poles (66.4194, 2.4111) (66.545, 2.561) (66.6746, 2.9581) (66.6746, 3.2255) knots 0 0 0 1 2 2 2
  spline S126 degree 2 poles (66.6746, 3.2255) (66.6746, 3.4929) (66.5288, 3.8333) (66.391, 3.9467) knots 0 0 0 1 2 2 2
  spline S127 degree 2 poles (66.391, 3.9467) (66.2492, 4.0723) (65.8278, 4.1777) (65.5725, 4.1777) knots 0 0 0 1 2 2 2
  spline S128 degree 2 poles (65.5725, 4.1777) (65.297, 4.1777) (64.75, 4.0926) (64.5839, 4.0561) knots 0 0 0 1 2 2 2
  line L181 (64.5839, 4.0561) -> (64.5839, 6.6331)
  line L182 (64.5839, 6.6331) -> (67.327, 6.6331)
  line L183 (67.327, 6.6331) -> (67.327, 6.0456)
  line L184 (67.327, 6.0456) -> (65.2281, 6.0456)
  line L185 (65.2281, 6.0456) -> (65.2281, 4.7125)
  spline S129 degree 2 poles (65.2281, 4.7125) (65.3497, 4.7287) (65.5847, 4.7409) (65.6819, 4.7409) knots 0 0 0 1 2 2 2
  spline S130 degree 2 poles (65.6819, 4.7409) (66.0669, 4.7409) (66.5977, 4.6153) (66.8408, 4.4289) knots 0 0 0 1 2 2 2
  spline S131 degree 2 poles (66.8408, 4.4289) (67.0879, 4.2425) (67.3554, 3.6752) (67.3554, 3.2214) knots 0 0 0 1 2 2 2
  point P0 (110, 0)
  constraints: 2 other
emboss "Emboss1" sketch "Sketch10" operation cut depth 1 direction (0, 0, -1)
body "Solid1"
